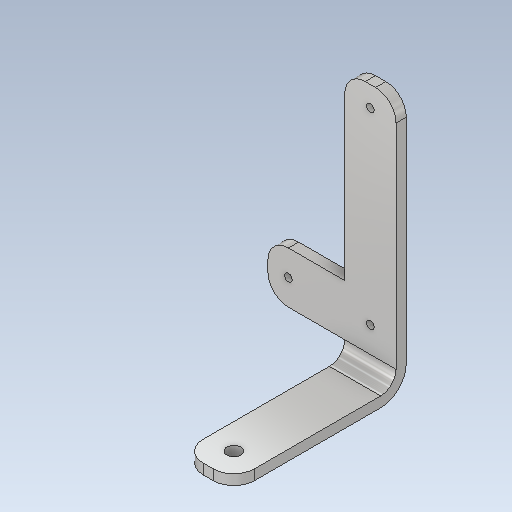
# Autodesk Inventor part: actuator_bracket2
Saved by Autodesk Inventor 2020 (Build 240168000, 168)
## iProperties
Created: 2017-11-30
Part Number: actuator_bracket2
Material: Generic
Document SubType Name: Modeling
Designer: stedrock
Density: 1 g/cm^3
Appearance: Default
Mass: 14.7792 g
Surface Area: 91.7827 cm^2
Volume: 14.7792 cm^3
Author: stedrock
Autodesk Inventor part; units mm, degrees
ref_plane "YZ Plane" through (0, 0, 0) normal (1, 0, 0) x (0, 1, 0)
ref_plane "XZ Plane" through (0, 0, 0) normal (0, 1, 0) x (-1, 0, 0)
ref_plane "XY Plane" through (0, 0, 0) normal (0, 0, 1) x (1, 0, 0)
sketch "Sketch1" plane through (0, 0, 0) normal (0, 0, 1) x (1, 0, 0)
  line L0 (0, 0) -> (20, 0)
  line L1 (20, 0) -> (20, 164.25)
  line L2 (20, 164.25) -> (0, 164.25)
  line L3 (0, 164.25) -> (0, 0)
  line L4 (0, 73) -> (-30, 73)
  line L5 (-30, 73) -> (-30, 93)
  line L6 (-30, 93) -> (0, 93)
  line L7 (0, 93) -> (0, 73)
  circle A0 centre (10, 10) radius 2.75
  line L8 (0, 73) -> (20, 73)
  circle A1 centre (-22, 83) radius 1.5
  circle A2 centre (10, 156.25) radius 1.5
  circle A3 centre (10, 83) radius 1.5
  dimension "d0" = 20
  dimension "d1" = 164.25
  dimension "d2" = 20
  dimension "d3" = 30
  dimension "d4" = 73
  dimension "d5" = 5.5
  dimension "d6" = 10
  dimension "d7" = 10
  dimension "d13" = 3
  dimension "d14" = 3
  dimension "d15" = 3
  dimension "d17" = 8
  dimension "d18" = 10
  dimension "d19" = 8
  dimension "d20" = 10
  dimension "d21" = 10
  dimension "d22" = 10
  constraints: 18 end point, 4 centre point, 4 parallel, 3 perpendicular, 2 horizontal, 2 point on line
  measures "d0" distance of L2.end L1.end
  measures "d1" distance of L1.end L0.end
  measures "d2" distance of L4.end L5.end
  measures "d3" distance of L4.start L4.end
  measures "d4" distance of L0.start L4.start
  measures "d5" diameter of A0
  measures "d6" distance from line of L3 A0.centre
  measures "d7" distance from line of L0 A0.centre
  measures "d13" diameter of A1
  measures "d14" diameter of A2
  measures "d15" diameter of A3
  measures "d17" distance from line of L5 A1.centre
  measures "d18" distance from line of L1 A2.centre
  measures "d19" distance from line of L2 A2.centre
  measures "d20" distance from line of L1 A3.centre
  measures "d21" distance from line of L4 A1.centre
  measures "d22" distance from line of L8 A3.centre
extrude "Extrusion1" add sketch "Sketch1" along normal blind 4
bend part "Bend Part1" radius 10 angle 90 line through (0, 73, 0) along (1, 0, 0) centre toward (0, 0, 1) moving side (0, -1, 0) both sides no
fillet "Fillet1" radius 8 6 edges at (-30, 73, 2) (-30, 93, 2) (0, 164.25, 2) (20, 164.25, 2) (0, 65, 67.292) (20, 65, 67.292)
equation "\"d1\" = 2.25 * d4"
equation "\"d6\" = 0.5 * d0"
equation "\"d14\" = d13"
equation "\"d15\" = d13"
equation "\"d18\" = 0.5 * d0"
equation "\"d20\" = 0.5 * d0"
equation "\"d21\" = 0.5 * d2"
equation "\"d22\" = d21"
body "Solid1"
